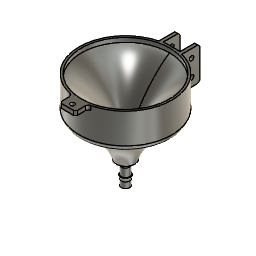
Holder_thing v13 (Autodesk Fusion 360 design; units mm, degrees)
Autodesk Fusion 360 part; units mm, degrees
note: some values were not read from the file. Chosen so that the rebuilt part matches the saved one: which face or edge a step refers to. Set by a fixed rule: which sketch regions a step uses.
sketch "Sketch1" plane through (0, 0, 0) normal (1, 0, 0) x (0, 1, 0)
  line L0 (0, 0) -> (0, 97.4344) construction
  line L1 (55.54, 97.4344) -> (55.54, 8.5344)
  line L2 (55.54, 8.5344) -> (6.909, 8.5344)
  line L3 (6.909, 8.5344) -> (6.909, 5.9944) construction
  line L4 (6.909, 5.9944) -> (9.449, 5.9944) construction
  line L5 (9.449, 5.9944) -> (9.449, 0) construction
  line L6 (9.449, 0) -> (4.75, 0) construction
  line L7 (4.75, 0) -> (4.75, 10.16) construction
  line L8 (4.75, 10.16) -> (3.5, 10.16) construction
  line L9 (3.5, 10.16) -> (3.5, 13.6144)
  line L10 (55.54, 97.4344) -> (53, 97.4344)
  spline S0 degree 5 poles (3.5, 13.6144) (3.5, 17.7131) (4.2042, 25.8255) (7.3712, 37.7389) (15.1289, 53.0255) (28.0111, 70.3516) (38.797, 81.6923) (46.2562, 88.013) (50.8203, 91.0959) (53, 92.3544) knots 0 0 0 0 0 0 0.2 0.4 0.6 0.8 1 1 1 1 1 1
  line L11 (47.5007, 89.1794) -> (58.4993, 95.5294)
  line L12 (3.5, 3.4544) -> (3.5, 23.7744)
  line L13 (55.54, 57.4344) -> (11.09, 8.5344) construction
  line L14 (53, 97.4344) -> (53, 92.3544)
  spline S1 degree 5 poles (11.09, 8.5344) (11.6891, 11.0199) (13.2478, 15.9064) (16.6662, 22.9835) (23.073, 31.9259) (33.0375, 42.147) (41.8287, 49.2525) (48.6266, 53.726) (53.2246, 56.2712) (55.54, 57.4344) knots 0 0 0 0 0 0 0.2 0.4 0.6 0.8 1 1 1 1 1 1
  line L15 (48.8884, 54.0928) -> (62.1916, 60.776)
  line L16 (9.4145, 1.5836) -> (12.7655, 15.4852)
  line L17 (3.5, 10.16) -> (3.5, -18.8956)
  line L18 (3.5, -18.8956) -> (5, -18.8956)
  line L19 (5.9, -7.4656) -> (5, -7.4656)
  line L20 (5, -7.4656) -> (5, 8.5344)
  line L21 (5, 8.5344) -> (6.909, 8.5344)
  line L22 (5, -18.8956) -> (5, -12.0376)
  line L23 (5, -12.0376) -> (5.9, -7.4656)
  point P0 (53, 97.4344)
  point P1 (55.54, 57.4344)
  dimension "d19" = 2.54
  dimension "d20" = 53
  dimension "d22" = 5.08
  dimension "d23" = 4.699
  dimension "d24" = 4.75
  dimension "d25" = 3.5
  dimension "d26" = 10.16
  dimension "d27" = 2.54
  dimension "d29" = 2.54
  dimension "d63" = 5.9944
  dimension "d92" = 88.9
  dimension "d96" = 30
  dimension "d98" = 20.32
  dimension "d99" = 12.7
  dimension "d101" = 40
  dimension "d106" = 44.45
  dimension "d112" = 5.08
  dimension "d130" = 1.5
  dimension "d131" = 2.4
  dimension "d132" = 16
  dimension "d133" = 1.5
  dimension "d134" = 11.43
  dimension "d135" = 6.858
  constraint coincident L0.start origin
  constraint vertical L0
  constraint parallel L0 L1
  constraint perpendicular L1 L2
  constraint perpendicular L2 L3
  constraint perpendicular L3 L4
  constraint perpendicular L2 L5
  constraint perpendicular L5 L6
  constraint perpendicular L6 L7
  constraint perpendicular L7 L8
  constraint perpendicular L6 L9
  constraint horizontal L1.start P0
  constraint horizontal L0.end P0
  constraint horizontal L0.start L6.end
  constraint midpoint S0.end L11
  constraint midpoint L9.end L12
  constraint vertical L12
  constraint coincident L1 P1
  constraint coincident P1 L13.start
  constraint coincident L2 L13.end
  constraint horizontal L10
  constraint vertical L14
  constraint midpoint P1 L15
  constraint midpoint L13.end L16
  constraint coincident P0 L10.end
  constraint perpendicular L8 L17
  constraint perpendicular L12 L18
  constraint perpendicular L2 L20
  constraint perpendicular L3 L21
  constraint horizontal L19
  constraint vertical L22
  measures "d19" distance of L1.start P0
  measures "d20" horizontal distance of L0.end P0
  measures "d22" vertical distance of L2.end L9.end
  measures "d23" distance of L5.end L6.end
  measures "d24" distance of L0.start L6.end
  measures "d25" horizontal distance of L0.start L8.end
  measures "d26" distance of L6.end L7.end
  measures "d27" horizontal distance of L2.end L4.end
  measures "d29" distance of L2.end L3.end
  measures "d63" distance of L4.end L5.end
  measures "d92" distance of L1.start L1.end
  measures "d96" angle of L2 L11
  measures "d98" distance of L12.start L12.end
  measures "d99" distance of L11.start L11.end
  measures "d101" distance of L1.start P1
  measures "d106" distance of L1.end L13.end
  measures "d112" distance of S0.end P0
  measures "d130" distance of L17.end L18.end
  measures "d131" distance of L17 L19.start
  measures "d132" distance of L19.end L20.end
  measures "d133" distance of L17 L20
  measures "d134" vertical distance of L18.end L19.start
  measures "d135" distance of L18.end L22.end
revolve "Revolve1" add sketch "Sketch1" angle 360 about axis through (0, 0, 0) along (0, 0, 1) contours L1 L2 L9 S0 L11 L12 S1 L17 L18 L19 L20 L21 L22 L23 | L1 L10 L11 L14
sketch "Sketch2" plane through (0, 0, 0) normal (0, 1, 0) x (1, 0, 0)
ref_plane "WorkPlane1" through (0, 55.54, 75.6249) normal (0, 1, 0) x (-1, 0, 0)
sketch "Sketch3" plane through (0, 55.54, 0) normal (0, 1, 0) x (1, 0, 0)
  line L0 (55.54, -97.4344) -> (-55.54, -97.4344)
  line L1 (13.81, -97.4344) -> (10, -97.4344)
  line L2 (10, -97.4344) -> (10, -57.4344)
  line L3 (10, -57.4344) -> (13.81, -57.4344)
  line L4 (13.81, -57.4344) -> (13.81, -97.4344)
  line L5 (-10, -97.4344) -> (-13.81, -97.4344)
  line L6 (-13.81, -97.4344) -> (-13.81, -57.4344)
  line L7 (-13.81, -57.4344) -> (-10, -57.4344)
  line L8 (-10, -57.4344) -> (-10, -97.4344)
  line L9 (10, -97.4344) -> (-10, -97.4344)
  dimension "d33" = 3.81
  dimension "d34" = 3.81
  dimension "d35" = 20
  dimension "d93" = 40
  constraint horizontal L1
  constraint vertical L2
  constraint horizontal L3
  constraint vertical L4
  constraint coincident L0 L1.start
  constraint horizontal L5
  constraint vertical L6
  constraint horizontal L7
  constraint vertical L8
  constraint coincident L0 L5.start
  constraint midpoint L0 L9
  constraint horizontal L2.end L7.end
  constraint coincident L6.end L7.start
  measures "d33" distance of L1.start L1.end
  measures "d34" distance of L5.start L5.end
  measures "d35" distance of L1.end L5.start
  measures "d93" distance of L5.end L6.end
extrude "Extrude2" add sketch "Sketch3" along normal blind 20 and the other way up to surface second end surface at (2.7684, 55.471, 96.2299)
sketch "Sketch4" plane through (0, 0, 97.4344) normal (0, 0, 1) x (-1, 0, 0)
  arc A0 (-10, -54.6323) -> (10, -54.6323) centre (0, 0) ccw
  line L0 (-10, -55.54) -> (10, -55.54)
  line L1 (-10, -54.6323) -> (-10, -75.54)
  line L2 (10, -54.6323) -> (10, -75.54)
extrude "Extrude3" add sketch "Sketch4" against normal blind 40
ref_plane "WorkPlane2" through (0, 65.0862, 77.4344) normal (1, 0, 0) x (0, 0, -1)
sketch "Sketch6" plane through (-13.81, 0, 0) normal (-1, 0, 0) x (0, -1, 0)
  line L0 (-75.54, 97.4344) -> (-75.54, 57.4344)
  line L1 (-53.7957, 97.4344) -> (-75.54, 97.4344)
  line L2 (-65.54, 97.4344) -> (-65.54, 87.4344)
  line L3 (-65.54, 87.4344) -> (-65.54, 67.4344)
  line L4 (-65.54, 67.4344) -> (-65.54, 57.4344)
  line L5 (-75.54, 87.4344) -> (-65.54, 87.4344) construction
  line L6 (-65.54, 87.4344) -> (-55.54, 87.4344) construction
  line L7 (-55.54, 97.4344) -> (-55.54, 57.4344)
  line L8 (-53.7957, 57.4344) -> (-75.54, 57.4344)
  point P0 (-55.54, 97.4344)
  dimension "d59" = 10
  dimension "d109" = 10
  constraint coincident L1 L2.start
  constraint perpendicular L1 L2
  constraint perpendicular L1 L3
  constraint coincident L0 L5.start
  constraint coincident L3 L2.end
  constraint perpendicular L3 L6
  constraint collinear L5 L6
  constraint equal L5 L6
  constraint coincident L6.end L7
  constraint collinear L3 L4
  constraint coincident L2.end L3.start
  constraint coincident L4.end L8
  measures "d59" distance of L2.start L2.end
  measures "d109" distance of L3.end L4.end
hole "Hole1" at (-13.81, 65.54, 87.4344) at (-13.81, 65.54, 67.4344) direction (1, 0, 0) diameter 5.5118 depth 30.48 tip angle 118
ref_plane "WorkPlane3" through (0, -9.449, 2.8733) normal (0, -1, 0) x (1, 0, 0)
sketch "Sketch7" plane through (0, -9.449, 0) normal (0, -1, 0) x (-1, 0, 0)
  line L0 (0, 0) -> (0.8, 0)
  line L1 (0.8, 0) -> (0.8, -7.62)
  line L2 (0.8, -7.62) -> (-0.8, -7.62)
  line L3 (-0.8, -7.62) -> (-0.8, 0)
  line L4 (-0.8, 0) -> (0, 0)
  dimension "d66" = 7.62
  dimension "d67" = 1.6
  constraint coincident L0.start L4.end
  constraint horizontal L0
  constraint perpendicular L0 L1
  constraint perpendicular L1 L2
  constraint perpendicular L2 L3
  constraint perpendicular L1 L4
  constraint equal L0 L4
  measures "d66" distance of L2.end L3.end
  measures "d67" distance of L0.end L3.end
extrude "Extrude5" [suppressed]
fillet "Fillet3" [suppressed]
sketch "Sketch8" plane through (0.8, 0, 0) normal (-1, 0, 0) x (0, -1, 0)
  line L0 (9.4151, 0) -> (4.6821, 0) construction
  line L1 (4.6821, 0) -> (4.6821, 5.9944) construction
  line L2 (4.6821, 5.9944) -> (9.4151, 5.9944) construction
  line L3 (9.4151, 5.9944) -> (9.4151, 0) construction
  line L4 (4.6821, 5.9944) -> (9.4151, 0) construction
  line L5 (4.6821, 0) -> (9.4151, 5.9944) construction
  point P0 (9.4151, 5.9944)
  point P1 (9.4151, 0)
  point P2 (4.6821, 0)
  point P3 (7.0486, 2.9972)
  constraint horizontal L0
  constraint vertical L1
  constraint horizontal L2
  constraint vertical L3
  constraint coincident P1 L0.start
  constraint coincident P0 L2.end
  constraint coincident P2 L0.end
  constraint midpoint L4 P3
hole "Hole2" [suppressed]
ref_plane "WorkPlane4" through (9.449, 0, 2.266) normal (1, 0, 0) x (0, 1, 0)
sketch "Sketch9" plane through (9.449, 0, 0) normal (1, 0, 0) x (0, 1, 0)
  circle A0 centre (-7.0486, 2.9972) radius 1.1938
  circle A1 centre (-7.0486, 2.9972) radius 2.2
  dimension "d76" = 4.4
  constraint concentric A0 A1
  measures "d76" diameter of A1
extrude "Extrude6" [suppressed]
hole "Hole3" [suppressed]
fillet "Fillet4" [suppressed]
fillet "Fillet5" [suppressed]
ref_plane "WorkPlane5" through (-9.449, 0, 3.1659) normal (-1, 0, 0) x (0, -1, 0)
sketch "Sketch10" plane through (-9.449, 0, 0) normal (-1, 0, 0) x (0, -1, 0)
  circle A0 centre (7.0486, 2.9972) radius 1.1938 construction
  line L0 (9.0986, 4.1808) -> (7.0486, 5.3643)
  line L1 (7.0486, 5.3643) -> (4.9986, 4.1808)
  line L2 (4.9986, 4.1808) -> (4.9986, 1.8136)
  line L3 (4.9986, 1.8136) -> (7.0486, 0.6301)
  line L4 (7.0486, 0.6301) -> (9.0986, 1.8136)
  line L5 (9.0986, 1.8136) -> (9.0986, 4.1808)
  point P0 (7.0486, 2.9972)
  dimension "d87" = 4.1
  constraint coincident P0 A0.centre
  constraint vertical L0.end P0
  measures "d87" distance of L2 L5
chamfer "Chamfer3" distance 2.54 angle 45 4 edges at (-11.905, 75.54, 97.4344) (-11.905, 75.54, 57.4344) (11.905, 75.54, 57.4344) (11.905, 75.54, 97.4344)
extrude "Extrude7" [suppressed]
sketch "Sketch11" plane through (0, 0, 97.4344) normal (0, 0, 1) x (-1, 0, 0)
  arc A0 (13.81, -53.7957) -> (-13.81, -53.7957) centre (0, 0) ccw
  line L0 (9.525, 54.7171) -> (9.525, 69.7171)
  line L1 (9.525, 69.7171) -> (-9.525, 69.7171)
  line L2 (-9.525, 69.7171) -> (-9.525, 54.7171)
  line L3 (0, 69.7171) -> (0, 0)
  point P0 (0, 63.7171)
  dimension "d113" = 19.05
  dimension "d114" = 15
  dimension "d122" = 6
  constraint coincident A0 L0.start
  constraint vertical L0
  constraint perpendicular L0 L1
  constraint coincident A0 L2.end
  constraint perpendicular L1 L2
  constraint midpoint L1 L3.start
  constraint coincident A0.centre L3.end
  constraint vertical L3
  constraint coincident L3 P0
  measures "d113" distance of L0.end L1.end
  measures "d114" distance of L1.end L2.end
  measures "d122" distance of L1 P0
extrude "Extrude8" add sketch "Sketch11" against normal blind 5.08
chamfer "Chamfer5" distance 2.54 angle 45 2 edges at (-9.525, -69.7171, 94.8944) (9.525, -69.7171, 94.8944)
fillet "Fillet8" radius 3.81 2 edges at (-9.525, -54.7171, 94.8944) (9.525, -54.7171, 94.8944)
hole "Hole4" at (0, -63.7171, 97.4344) direction (0, 0, -1) diameter 5.5118 depth 12.7 tip angle 118
fillet "Fillet9" radius 6.35 1 edges at (0, -55.54, 57.4344)
chamfer "Chamfer6" distance 6.09 angle 45 1 edges at (-4.6616, 1.8081, 8.5344)
ref_plane "WorkPlane6" through (-55.54, 0, 75.3331) normal (-1, 0, 0) x (0, -1, 0)
sketch "Sketch13" plane through (-55.54, 0, 0) normal (-1, 0, 0) x (0, -1, 0)
  line L0 (-53.7957, 61.2503) -> (55.54, 61.2503)
  line L1 (-53.7957, 61.2503) -> (-53.7957, 97.4344)
  line L2 (-53.7957, 97.4344) -> (54.1199, 97.4344)
  line L3 (54.1199, 97.4344) -> (54.1199, 92.3544)
  line L4 (54.1199, 92.3544) -> (55.54, 92.3544)
  line L5 (54.1199, 92.3544) -> (54.1199, 97.4344)
  line L6 (-53.7957, 97.4344) -> (54.1199, 97.4344)
  line L7 (-53.7957, 97.4344) -> (-53.7957, 61.2503)
  line L8 (0, 97.4344) -> (0, 69.4944)
  line L9 (0, 69.4944) -> (0, 61.2503)
  point P0 (0, 97.4344)
  point P1 (0, 69.4944)
  dimension "d138" = 27.94
  constraint coincident P0 L8.start
  constraint perpendicular L2 L8
  constraint coincident L0 L9.end
  constraint perpendicular L0 L9
  constraint coincident P1 L8.end
  measures "d138" distance of P0 P1
sketch "Sketch14" plane through (0, 0, 0) normal (0, 1, 0) x (1, 0, 0)
  spline S0 degree 3 poles (-55.54, -65.9944) (-55.54, -65.9944) (-55.5342, -66.0823) (-55.5134, -66.4395) (-55.4987, -66.7088) (-55.471, -67.3302) (-55.4562, -67.7237) (-55.4354, -68.586) (-55.4296, -69.0548) (-55.4296, -69.934) (-55.4354, -70.4028) (-55.4562, -71.2651) (-55.471, -71.6586) (-55.4987, -72.28) (-55.5134, -72.5493) (-55.5342, -72.9065) (-55.54, -72.9944) (-55.54, -72.9944) knots 0.527511 0.527511 0.527511 0.527511 0.659389 0.659389 0.791267 0.791267 0.923145 0.923145 1.055023 1.055023 1.186901 1.186901 1.318778 1.318778 1.450656 1.450656 1.582534 1.582534 1.582534 1.582534
  spline S1 degree 3 poles (-55.54, -72.9944) (-55.54, -72.9944) (-55.5342, -72.9065) (-55.5134, -72.5493) (-55.4987, -72.28) (-55.471, -71.6586) (-55.4562, -71.2651) (-55.4354, -70.4028) (-55.4296, -69.934) (-55.4296, -69.4944) (-55.4296, -69.0548) (-55.4354, -68.586) (-55.4562, -67.7237) (-55.471, -67.3302) (-55.4987, -66.7088) (-55.5134, -66.4395) (-55.5342, -66.0823) (-55.54, -65.9944) (-55.54, -65.9944) knots 1.582534 1.582534 1.582534 1.582534 1.714412 1.714412 1.84629 1.84629 1.978167 1.978167 2.110045 2.110045 2.110045 2.241923 2.241923 2.373801 2.373801 2.505679 2.505679 2.637557 2.637557 2.637557 2.637557
  line L0 (-53, -74.4944) -> (-70.54, -74.4944) construction
  line L1 (-70.54, -74.4944) -> (-70.54, -75.3944) construction
  line L2 (-81.97, -74.4944) -> (-81.97, -72.9944) construction
  line L3 (-81.97, -72.9944) -> (-53, -72.9944) construction
  line L4 (-53, -72.9944) -> (-53, -74.4944) construction
  line L5 (-55.54, -72.9944) -> (-55.54, -69.4944) construction
  line L6 (-55.54, -69.4944) -> (-55.54, -65.9944) construction
  line L7 (-55.54, -69.4944) -> (-70.0195, -69.4944) construction
  line L8 (-70.54, -75.3944) -> (-75.112, -74.4944) construction
  line L9 (-75.112, -74.4944) -> (-81.97, -74.4944) construction
  line L10 (0, -97.4344) -> (0, -88.8544)
  line L11 (55.54, -76.1544) -> (70.0195, -76.1544) construction
  line L12 (53, -81.1544) -> (70.54, -81.1544)
  line L13 (70.54, -82.0544) -> (75.112, -81.1544)
  line L14 (81.97, -79.6544) -> (53, -79.6544)
  line L15 (53, -79.6544) -> (53, -81.1544)
  line L16 (55.54, -79.6544) -> (55.54, -65.8067) construction
  line L17 (70.54, -81.1544) -> (70.54, -82.0544)
  line L18 (55.54, -65.8067) -> (55.54, -76.1544) construction
  line L19 (81.97, -81.1544) -> (81.97, -79.6544)
  line L20 (75.112, -81.1544) -> (81.97, -81.1544)
  point P0 (-55.54, -69.4944)
  point P1 (0, -97.4344)
  point P2 (46.65, -76.1544)
  point P3 (55.54, -97.4344)
  dimension "d142" = 5
  dimension "d143" = 3.5
  dimension "d144" = 5.9
  dimension "d145" = 6.858
  dimension "d146" = 4.572
  dimension "d147" = 15
  dimension "d148" = 2.54
  dimension "d161" = 6.858
  dimension "d162" = 17.54
  dimension "d163" = 28.97
  dimension "d164" = 3.5
  dimension "d165" = 5
  dimension "d166" = 5
  dimension "d167" = 5.9
  dimension "d168" = 4.572
  dimension "d169" = 53
  dimension "d170" = 4.6597
  dimension "d172" = 8.89
  dimension "d173" = 12.7
  dimension "d174" = 17.78
  constraint horizontal L0
  constraint perpendicular L0 L1
  constraint parallel L1 L2
  constraint perpendicular L2 L3
  constraint vertical L4
  constraint coincident S0.end S1.start
  constraint coincident S0.start S1.end
  constraint equal L5 L6
  constraint collinear L5 L6
  constraint coincident P0 L5.end
  constraint perpendicular L6 L7
  constraint horizontal L9
  constraint collinear L0 L9
  constraint coincident P1 L10.start
  constraint vertical L10
  constraint vertical L18
  constraint perpendicular L14 L16
  constraint coincident L16.start L14
  constraint horizontal L20
  constraint horizontal L12
  constraint horizontal L14
  constraint vertical L17
  constraint vertical L19
  constraint coincident L11.start L18
  constraint horizontal P2 L11.start
  constraint vertical L16.start P3
  measures "d142" distance of L0 L7
  measures "d143" distance of L3 L7
  measures "d144" distance of L1.end L7
  measures "d145" distance of L2.start L8.end
  measures "d146" horizontal distance of L1.end L8.end
  measures "d147" distance of L0.end S0.end
  measures "d148" distance of L0.start S0.end
  measures "d161" distance of L19.start L13.end
  measures "d162" distance of L12.start L12.end
  measures "d163" distance of L14.end L14.start
  measures "d164" distance of L11 L14
  measures "d165" distance of L19.start L11
  measures "d166" vertical distance of P2 L12.start
  measures "d167" vertical distance of P2 L13.start
  measures "d168" horizontal distance of L13.end L13.start
  measures "d169" horizontal distance of L10.end L14.end
  measures "d170" distance of L13.end L13.start
  measures "d172" distance of P2 L11.start
  measures "d173" vertical distance of L10.end L11.start
  measures "d174" distance of L16.start P3
revolve "Revolve3" [suppressed]
sketch "Sketch15" plane through (81.97, 0, 0) normal (1, 0, 0) x (0, 1, 0)
  point P0 (0, 76.1544)
hole "Hole6" [suppressed]
fillet "Fillet12" [suppressed]
chamfer "Chamfer8" [suppressed]
equation "d131 = 11.8 mm / 2 - 3.5 mm"
equation "d144 = 11.8 mm / 2"
